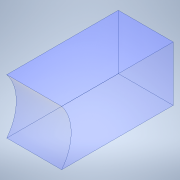
# Autodesk Inventor part: shank_2
Saved by Autodesk Inventor 2020.2 (Build 242310000, 310)
## iProperties
Created: 2021-01-30
Part Number: shank_2
Material: Generic
Document SubType Name: Modeling
Designer: DELL
Density: 1 g/cm^3
Appearance: Clear - Blue
Author: DELL
Autodesk Inventor part; units mm, degrees
ref_plane "YZ Plane" through (0, 0, 0) normal (1, 0, 0) x (0, 1, 0)
ref_plane "XZ Plane" through (0, 0, 0) normal (0, 1, 0) x (-1, 0, 0)
ref_plane "UCS1: YZ Plane" through (0, 0, 0) normal (1, 0, 0) x (0, 1, 0)
sketch "Sketch11" plane through (0, 0, 0) normal (1, 0, 0) x (0, 1, 0)
  line L0 (-67.9, 0) -> (67.9, 0) construction
  line L1 (0, -249.7) -> (0, 98.2) construction
  circle A0 centre (0, 0) radius 32.5
  circle A1 centre (0, 0) radius 48.5
  line L2 (-30, -38.1084) -> (-30, -160)
  line L3 (-30, -160) -> (30, -160)
  line L4 (30, -160) -> (30, -38.1084)
  dimension "d77" = 65
  dimension "d78" = 97
  dimension "d79" = 60
  dimension "d80" = 160
  constraints: 6 end point, 2 centre point, 2 coincident, 2 perpendicular, 2 point on circle, 1 vertical, 1 other
  measures "d77" diameter of A0
  measures "d78" diameter of A1
  measures "d79" distance between parallel lines of L4 L2
  measures "d80" distance from line of L3.end L0
extrude "Extrusion11" add sketch "Sketch11" along normal mid plane 60 contours A1 L4 L3 L2
sketch "Sketch6" plane through (0, 0, 0) normal (1, 0, 0) x (0, 1, 0)
  circle A0 centre (0, 0) radius 32.5
  line L0 (-32.5, 0) -> (-32.5, -80)
  line L1 (-32.5, -80) -> (32.5, -80)
  line L2 (32.5, -80) -> (32.5, 0)
  line L3 (0, 0) -> (0, -80) construction
  line L4 (-32.5, -60) -> (32.5, -60)
  circle A1 centre (0, 0) radius 48.5
  point P0 (32.5, -36)
  point P1 (23.3184, -32.5)
  point P2 (0, -40)
  point P3 (-32.5, -36)
  dimension "d38" = 65
  dimension "d39" = 80
  dimension "d74" = 97
  dimension "d75" = 20
  dimension "d48" = 10
  dimension "d73" = 55
  dimension "d52" = 120
  constraints: 2 end point, 1 midpoint, 1 vertical
  measures "d52" distance from line of L0 L1.end
sketch "Sketch5" plane through (0, 0, -171) normal (0, 0, -1) x (-1, 0, 0)
  circle A0 centre (0, 0) radius 10
  point P0 (0, 0)
  dimension "d35" = 20
  constraints: 1 centre point, 1 coincident
  measures "d35" diameter of A0
body "Solid1"
body "Solid4"
body "Solid5"
